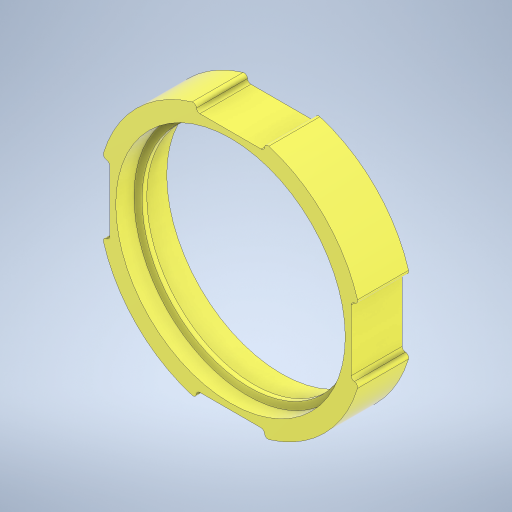
# Autodesk Inventor part: rosca_2
Saved by Autodesk Inventor 2023.2 (Build 272271030, 271C)
## iProperties
Created: 2023-10-23
Part Number: rosca_2
Material: Generic
Document SubType Name: Modeling
Designer: Cris Pat
Density: 1 g/cm^3
Appearance: Default
Author: Cris Pat
Autodesk Inventor part; units mm, degrees
ref_plane "YZ Plane" through (0, 0, 0) normal (1, 0, 0) x (0, 1, 0)
ref_plane "XZ Plane" through (0, 0, 0) normal (0, 1, 0) x (-1, 0, 0)
ref_plane "XY Plane" through (0, 0, 0) normal (0, 0, 1) x (1, 0, 0)
sketch "Sketch1" plane through (0, 0, 0) normal (0, 0, 1) x (1, 0, 0)
  circle A0 centre (0, 0) radius 31.2225
  dimension "d0" = 62.445
  constraints: 1 centre point, 1 coincident
  measures "d0" diameter of A0
extrude "Extrusion1" add sketch "Sketch1" against normal blind 12
sketch "Sketch2" plane through (0, 0, 0) normal (0, 0, 1) x (1, 0, 0)
  circle A0 centre (0, 0) radius 27
  dimension "d3" = 54
  constraints: 1 centre point, 1 coincident
  measures "d3" diameter of A0
extrude "Extrusion2" cut sketch "Sketch2" against normal through all
sketch "Sketch3" plane through (0, 0, 0) normal (1, 0, 0) x (0, 1, 0)
  line L0 (27, 0) -> (27, -12) construction
  line L1 (27, -12) -> (-27, -12) construction
  line L2 (27, -5.056) -> (27, -6.944)
  line L3 (27, -6.944) -> (25.5, -6.556)
  line L4 (25.5, -6.556) -> (25.5, -5.444)
  line L5 (25.5, -5.444) -> (27, -5.056)
  line L6 (-27, 0) -> (27, 0) construction
  point P0 (0, 0)
  point P1 (26.25, -6.75)
  point P2 (26.25, -5.25)
  point P3 (25.5, -6)
  dimension "d6" = 1.5
  dimension "d7" = 1.5
  dimension "d8" = 75.5
  dimension "d9" = 6
  constraints: 8 end point, 3 midpoint, 1 equal length, 1 parallel, 1 vertical, 1 vertical alignment
  measures "d6" distance between parallel lines of L4 L2
  measures "d7" distance of point (26.25, -6.75) point (26.25, -5.25)
  measures "d8" angle of L3 L2
  measures "d9" distance from line of L6 point (25.5, -6)
coil "Coil1" sketch "Sketch3" operation add axis through (0, 0, -10) along (0, 0, 1) pitch 3 turns 1 hand right
chamfer "Chamfer1" distance 0.7 angle 45 4 edges at (0, 26.25, -2.25) (0, 26.25, -5.25) (0, 26.25, -3.75) (0, 26.25, -6.75)
sketch "Sketch4" plane through (0, 0, 0) normal (0, 0, 1) x (1, 0, 0)
  circle A0 centre (0, 0) radius 29.5 construction
  line L0 (-8, 31.2225) -> (8, 31.2225)
  line L1 (8, 31.2225) -> (8, 28.3945)
  line L2 (8, 28.3945) -> (-8, 28.3945)
  line L3 (-8, 28.3945) -> (-8, 31.2225)
  circle A1 centre (0, 0) radius 31.2225 construction
  point P0 (0, 31.2225)
  dimension "d21" = 59
  dimension "d22" = 16
  constraints: 8 end point, 2 parallel, 1 coincident, 1 horizontal, 1 midpoint, 1 perpendicular, 1 tangent, 1 vertical alignment, 3 other
  measures "d22" distance between parallel lines of L1 L3
extrude "Extrusion3" cut sketch "Sketch4" against normal through all
fillet "Fillet1" radius 0.8 4 edges at (-8, 28.3945, -6) (-8, 30.1802, -6) (8, 30.1802, -6) (8, 28.3945, -6)
pattern_circular "Circular Pattern1" count 4 over 360 about axis through (0, 0, -10) along (0, 0, 1) of "Fillet1", "Extrusion3"
sketch "Sketch5" plane through (0, 0, -12) normal (0, 0, -1) x (-1, 0, 0)
  line L0 (7.2, 28.3945) -> (-7.2016, 28.3945) construction
  arc A0 (1, 28.3945) -> (-1, 28.3945) centre (0, 28.3945) ccw
  line L1 (1, 28.3945) -> (-1, 28.3945)
  line L2 (7.2016, -28.3945) -> (-7.2, -28.3945) construction
  arc A1 (-1, -28.3945) -> (1, -28.3945) centre (0, -28.3945) ccw
  line L3 (1, -28.3945) -> (-1, -28.3945)
  point P0 (0, 0)
  dimension "d29" = 1
  dimension "d33" = 1
  constraints: 5 point on line, 4 end point, 4 point on circle, 2 centre point, 2 vertical alignment, 1 collinear, 1 horizontal, 1 horizontal alignment
  measures "d29" radius of A0
  measures "d33" radius of A1
extrude "Extrusion4" add sketch "Sketch5" against normal blind 5 contours L3 A1
fillet "Fillet2" radius 0.8 2 edges at (1, -28.3945, -9.5) (-1, -28.3945, -9.5)
body "Solid1"
